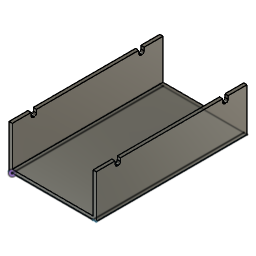
Cover (Autodesk Fusion 360 design; units mm, degrees)
part number: 2025-10-18-14-32-01-691
Autodesk Fusion 360 part; units mm, degrees
sketch "Sketch1" plane through (0, 0, 0) normal (0, 0, 1) x (1, 0, 0)
  line L0 (0, 0) -> (75, 0)
  line L1 (75, 0) -> (75, 140)
  line L2 (75, 140) -> (0, 140)
  line L3 (0, 140) -> (0, 0)
  line L4 (0, 140) -> (-3, 140)
  line L5 (-3, 140) -> (-3, 0)
  line L6 (-3, 0) -> (0, 0)
  line L7 (0, 0) -> (0, 140)
  line L8 (75, 140) -> (78, 140)
  line L9 (78, 140) -> (78, 0)
  line L10 (78, 0) -> (75, 0)
  line L11 (75, 0) -> (75, 140)
  dimension "d1" = 140
  dimension "d2" = 75
  dimension "d3" = 3
  dimension "d4" = 3
  constraint horizontal L0
  constraint vertical L1
  constraint horizontal L2
  constraint vertical L3
  constraint coincident L0.start L3.end
  constraint horizontal L4
  constraint vertical L5
  constraint horizontal L6
  constraint vertical L7
  constraint horizontal L8
  constraint vertical L9
  constraint horizontal L10
  constraint vertical L11
  measures "d1" distance of L0.start L2.end
  measures "d2" distance of L1 L3
  measures "d3" distance of L5 L7
  measures "d4" distance of L9 L11
extrude "Extrude1" add sketch "Sketch1" along normal blind 3 contours L0 L1 L2 L3 L7 L11
sketch "Sketch2" plane through (0, 0, 0) normal (0, 0, 1) x (1, 0, 0)
extrude "Extrude2" add sketch "Sketch1" along normal blind 40 contours L3 L4 L5 L6 L7 | L1 L8 L9 L10 L11
sketch "Sketch3" plane through (78, 0, 0) normal (1, 0, 0) x (0, 1, 0)
  line L0 (0, 0) -> (140, 0)
  line L1 (140, 0) -> (140, 40)
  line L2 (140, 40) -> (0, 40)
  line L3 (0, 40) -> (0, 0)
  line L4 (140, 0) -> (0, 0)
  line L5 (70, 40) -> (70, 0) construction
  line L6 (17.5, 40) -> (22.5, 40)
  line L7 (22.5, 40) -> (22.5, 37)
  line L8 (20.5, 35) -> (19.5, 35)
  line L9 (17.5, 37) -> (17.5, 40)
  arc A0 (17.5, 37) -> (19.5, 35) centre (19.5, 37) ccw
  arc A1 (20.5, 35) -> (22.5, 37) centre (20.5, 37) ccw
  line L10 (20, 40) -> (20, 35) construction
  line L11 (117.5, 40) -> (122.5, 40)
  line L12 (122.5, 40) -> (122.5, 37)
  line L13 (120.5, 35) -> (119.5, 35)
  line L14 (117.5, 37) -> (117.5, 40)
  arc A2 (117.5, 37) -> (119.5, 35) centre (119.5, 37) ccw
  arc A3 (120.5, 35) -> (122.5, 37) centre (120.5, 37) ccw
  line L15 (120, 35) -> (120, 40) construction
  point P0 (17.5, 35)
  point P1 (117.5, 35)
  dimension "d18" = 5
  dimension "d19" = 5
  dimension "d20" = 2
  dimension "d21" = 2
  dimension "d23" = 5
  dimension "d24" = 2
  dimension "d25" = 2
  dimension "d26" = 5
  dimension "d27" = 100
  constraint midpoint L2 L5.start
  constraint midpoint L4 L5.end
  constraint horizontal L6
  constraint vertical L7
  constraint horizontal L8
  constraint vertical L9
  constraint coincident L2 L6.start
  constraint coincident P0 L8
  constraint coincident P0 L9
  constraint tangent L8 A0
  constraint tangent L9 A0
  constraint tangent L7 A1
  constraint tangent L8 A1
  constraint midpoint L6 L10.start
  constraint midpoint L8 L10.end
  constraint horizontal L11
  constraint vertical L12
  constraint horizontal L13
  constraint vertical L14
  constraint coincident L2 L11.start
  constraint coincident P1 L13
  constraint coincident P1 L14
  constraint tangent L13 A2
  constraint tangent L14 A2
  constraint tangent L12 A3
  constraint tangent L13 A3
  constraint midpoint L13 L15.start
  constraint midpoint L11 L15.end
  constraint symmetric L5 L10 L15
  measures "d18" distance of L6.start P0
  measures "d19" distance of L7 L9
  measures "d20" radius of A0
  measures "d21" radius of A1
  measures "d23" distance of L12 L14
  measures "d24" radius of A2
  measures "d25" radius of A3
  measures "d26" distance of L11 L13
  measures "d27" distance of L10 L15
extrude "Extrude3" cut sketch "Sketch3" along normal mid plane 200 contours L2 L6 L7 L8 L9 A0 A1 | L2 L11 L12 L13 L14 A2 A3
